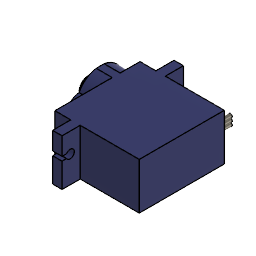
Dhanip_servo-final (Autodesk Fusion 360 design; units mm, degrees)
Autodesk Fusion 360 part; units mm, degrees
note: some values were not read from the file. Set by a fixed rule: which sketch regions a step uses.
sketch "Sketch1" plane through (0, 0, 0) normal (0, 0, 1) x (1, 0, 0)
  line L0 (11.15, -11.25) -> (-11.15, -11.25)
  line L1 (-11.15, -11.25) -> (-11.15, 11.25)
  line L2 (-11.15, 11.25) -> (11.15, 11.25)
  line L3 (11.15, 11.25) -> (11.15, -11.25)
  line L4 (11.15, -11.25) -> (-11.15, 11.25) construction
  line L5 (-11.15, -11.25) -> (11.15, 11.25) construction
  dimension "d1" = 22.3
  dimension "d2" = 22.5
  constraint horizontal L0
  constraint perpendicular L0 L1
  constraint parallel L0 L2
  constraint parallel L1 L3
  constraint coincident L4 origin
  constraint coincident L5 origin
  measures "d1" distance of L1.end L2.end
  measures "d2" distance of L0.end L1.end
extrude "Extrude1" add sketch "Sketch1" along normal blind 12.3 makes body 1
sketch "Sketch2" plane through (0, 0, 12.3) normal (0, 0, 1) x (-1, 0, 0)
  line L0 (-11.15, -11.25) -> (11.15, -11.25)
  line L1 (11.15, -11.25) -> (11.15, 11.25)
  line L2 (11.15, 11.25) -> (-11.15, 11.25)
  line L3 (-11.15, 11.25) -> (-11.15, -11.25)
  line L4 (11.15, -11.25) -> (6.95, -11.25)
  line L5 (6.95, -11.25) -> (6.95, -16.05)
  line L6 (6.95, -16.05) -> (4.45, -16.05)
  line L7 (4.45, -16.05) -> (4.45, -11.25)
  dimension "d5" = 4.2
  dimension "d6" = 4.8
  dimension "d7" = 2.5
  constraint coincident L0.end L1.start
  constraint perpendicular L1 L4
  constraint perpendicular L4 L5
  constraint perpendicular L5 L6
  constraint coincident L0 L7.end
  constraint perpendicular L0 L7
  measures "d5" distance of L0.end L4.end
  measures "d6" distance of L4.end L5.end
  measures "d7" distance of L5.end L6.end
extrude "Extrude2" add sketch "Sketch2" against normal blind 12.3 contours L0 L5 L6 L7 bodies 1
sketch "Sketch3" plane through (-4.45, 0, 0) normal (1, 0, 0) x (0, 1, 0)
  line L0 (16.05, 12.3) -> (11.25, 12.3)
  line L1 (11.25, 12.3) -> (11.25, 0)
  line L2 (11.25, 0) -> (16.05, 0)
  line L3 (16.05, 0) -> (16.05, 12.3)
  line L4 (16.05, 12.3) -> (16.05, 7.8)
  line L5 (16.05, 7.8) -> (14.86, 7.8)
  line L6 (14.86, 7.8) -> (14.86, 6.7)
  line L7 (14.86, 6.7) -> (16.05, 6.7)
  circle A0 centre (14.28, 7.25) radius 0.7993
  circle A1 centre (14.28, 7.25) radius 1.096
  dimension "d10" = 4.5
  dimension "d11" = 1.19
  dimension "d12" = 1.1
  dimension "d13" = 2.192
  constraint coincident L0.start L3.end
  constraint perpendicular L0 L4
  constraint perpendicular L4 L5
  constraint perpendicular L5 L6
  constraint coincident L3 L7.end
  constraint perpendicular L3 L7
  constraint coincident L5.end A0
  constraint concentric A0 A1
  measures "d10" distance of L0.start L4.end
  measures "d11" distance of L4.end L5.end
  measures "d12" distance of L5.end L6.end
  measures "d13" diameter of A1
extrude "Extrude3" cut sketch "Sketch3" against normal blind 2.5 contours L3 L5 L7 A1 | L5 L7 A0 A1 | L5 L7 A0 A1 | L6 A0 | L6 A0 bodies 1
mirror "Mirror1" about plane through (0, 0, 0) normal (0, 1, 0) of bodies 1 merged
sketch "Sketch4" plane through (-11.15, 0, 0) normal (-1, 0, 0) x (0, -1, 0)
  line L0 (-11.25, 0) -> (11.25, 0)
  line L1 (11.25, 0) -> (11.25, 12.3)
  line L2 (11.25, 12.3) -> (-11.25, 12.3)
  line L3 (-11.25, 12.3) -> (-11.25, 0)
  circle A0 centre (-4.953, 6.15) radius 6.2385
  line L4 (-4.73, 6.15) -> (0.611, 6.15)
  line L5 (0.611, 3.3285) -> (0.611, 9)
  circle A1 centre (0.611, 6.1643) radius 2.8357
  dimension "d18" = 5.341
  constraint horizontal L4
  constraint coincident A0 L5.start
  constraint perpendicular L4 L5
  constraint coincident L5.end A1
  constraint coincident L5.start A1
  measures "d18" distance of L4.start L4.end
extrude "Extrude4" add sketch "Sketch4" along normal blind 4.25 contours L0 L2 A0 A1 | A0 L5 | L4 L5 A1 | A0 L5 A1 | A0 L4 L5 A1 picked at (1.9534, 5.645) bodies 1
sketch "Sketch5" plane through (-15.4, 0, 0) normal (-1, 0, 0) x (0, -1, 0)
  arc A0 (0.611, 8.9715) -> (-3.9059, 12.3) centre (-4.953, 6.15) ccw
  line L0 (-3.9059, 12.3) -> (-6, 12.3)
  arc A1 (-6, 12.3) -> (-6, 0) centre (-4.953, 6.15) ccw
  line L1 (-6, 0) -> (-3.9059, 0)
  arc A2 (-3.9059, 0) -> (0.611, 3.3285) centre (-4.953, 6.15) ccw
  arc A3 (0.611, 3.3285) -> (0.611, 9) centre (0.611, 6.1643) ccw
  line L2 (0.611, 9) -> (0.611, 8.9715)
  line L3 (-0.4457, 1.8368) -> (-9.6223, 10.2871)
  line L4 (-0.2836, 10.2871) -> (-9.6223, 2.0129)
  circle A4 centre (-4.953, 6.15) radius 0.8
  circle A5 centre (-4.953, 6.15) radius 2.25
  dimension "d21" = 1.6
  dimension "d22" = 4.5
  constraint coincident A2 L3.start
  constraint coincident A1 L3.end
  constraint coincident A0 L4.start
  constraint coincident A1 L4.end
  constraint concentric A0 A4
  constraint concentric A4 A5
  measures "d21" diameter of A4
  measures "d22" diameter of A5
extrude "Extrude5" add sketch "Sketch5" along normal blind 3.1 contours L3 L4 A4 A5 | L3 L4 A4 A5 | L3 L4 A4 A5 | L3 L4 A4 A5 bodies 1
sketch "Sketch6" plane through (-18.5, 0, 0) normal (-1, 0, 0) x (0, -1, 0)
  circle A0 centre (-4.953, 6.15) radius 0.8
  circle A1 centre (-4.953, 6.15) radius 2.25
  line L0 (-3.3359, 4.5855) -> (-6.737, 7.5211)
  line L1 (-3.169, 7.5211) -> (-6.737, 4.7789)
  line L2 (-3.0017, 5.0296) -> (-2.8256, 4.8666)
  line L3 (-2.8256, 4.8666) -> (-2.992, 4.6868)
  line L4 (-2.992, 4.6868) -> (-3.1707, 4.7767)
  line L5 (-2.8256, 4.8666) -> (-2.9452, 5.1345)
  dimension "d25" = 0.24
  dimension "d26" = 0.245
  constraint coincident A1 L0.start
  constraint coincident A1 L0.end
  constraint coincident A1 L1.start
  constraint coincident A1 L1.end
  constraint coincident A1 L2.start
  constraint perpendicular L2 L3
  constraint coincident A1 L4.end
  constraint coincident A1 L5.end
  measures "d25" distance of L2.start L2.end
  measures "d26" distance of L2.end L3.end
extrude "Extrude6" add sketch "Sketch6" against normal blind 3.1 contours A1 L2 L3 L4 | A1 L2 L5 bodies 1
pattern_circular "C-Pattern1" count 40 over 360 about axis through (-15.4, 4.953, 6.15) along (-1, 0, 0) of "Extrude6"
sketch "Sketch7" plane through (0, 11.25, 0) normal (0, 1, 0) x (-1, 0, 0)
  line L0 (4.45, 0) -> (4.45, 12.3)
  line L1 (4.45, 12.3) -> (-11.15, 12.3)
  line L2 (-11.15, 12.3) -> (-11.15, 0)
  line L3 (-11.15, 0) -> (4.45, 0)
  line L4 (-11.15, 0) -> (-11.15, 3.88)
  line L5 (-11.15, 3.88) -> (-6.735, 3.88)
  circle A0 centre (-6.735, 3.88) radius 0.5
  circle A1 centre (-6.7332, 4.88) radius 0.5
  circle A2 centre (-6.7352, 5.88) radius 0.5
  dimension "d31" = 3.88
  dimension "d32" = 4.415
  dimension "d33" = 1
  dimension "d34" = 1
  dimension "d35" = 1
  constraint coincident L2.end L3.start
  constraint perpendicular L3 L4
  constraint perpendicular L4 L5
  constraint coincident L5.end A0.centre
  measures "d31" distance of L2.end L4.end
  measures "d32" distance of L4.end L5.end
  measures "d33" diameter of A0
  measures "d34" diameter of A1
  measures "d35" diameter of A2
extrude "Extrude7" add sketch "Sketch7" along normal blind 6 separate body contours A0 | A2 | A1 makes body 2 at (7.2344, 13.25, 3.8551)
extrude "Extrude8" add 1 faces at (-5.2833, 15.776, 7.8) along direction (0, 0, -1) blind 1.5 on bodies 1 bodies 1
extrude "Extrude9" add 1 faces at (-5.2833, 16.05, 8.2) along direction (0, -1, 0) blind 32.1 on bodies 1 bodies 1
sketch "Sketch9" plane through (-6.95, 0, 0) normal (-1, 0, 0) x (0, -1, 0)
  line L0 (-16.05, 12.3) -> (-16.05, 0)
  line L1 (-16.05, 0) -> (-11.25, 0)
  line L2 (-11.25, 0) -> (-11.25, 12.3)
  line L3 (-11.25, 12.3) -> (-16.05, 12.3)
  line L4 (-16.05, 12.3) -> (-16.05, 7.6)
  line L5 (-16.05, 7.6) -> (-16.05, 6.5)
  line L6 (-16.05, 7.6) -> (-16.05, 7.05)
  line L7 (-16.05, 7.05) -> (-13.898, 7.05)
  circle A0 centre (-13.898, 7.05) radius 1.1015
  line L8 (-16.05, 7.6) -> (-14.8524, 7.6)
  line L9 (-16.05, 6.5) -> (-14.8524, 6.5)
  point P0 (-24.3168, 27.9766)
  point P1 (-24.3168, 28.5266)
  dimension "d43" = 4.7
  dimension "d44" = 1.1
  dimension "d45" = 0.55
  dimension "d46" = 0.55
  dimension "d47" = 2.152
  dimension "d48" = 2.203
  constraint vertical L4
  constraint coincident L0.start L3.end
  constraint vertical L5
  constraint parallel L5 L6
  constraint perpendicular L6 L7
  constraint coincident L7.end A0.centre
  constraint coincident A0 L8.end
  constraint perpendicular L4 L8
  constraint coincident A0 L9.end
  constraint perpendicular L5 L9
  measures "d43" distance of L0.start L4.end
  measures "d44" distance of L4.end L5.end
  measures "d45" distance of P0 P1
  measures "d46" distance of L4.end L6.end
  measures "d47" distance of L6.end L7.end
  measures "d48" diameter of A0
extrude "Extrude10" cut sketch "Sketch9" against normal blind 2.5 contours L0 L5 L6 L7 A0 L8 | L0 L5 L7 A0 L9 | A0 bodies 1
mirror "Mirror2" about plane through (0, 0, 0) normal (0, 1, 0) of "Extrude10"
